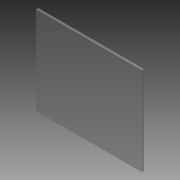
# Autodesk Inventor part: Wheel Shields
Saved by Autodesk Inventor 2013 (Build 170138000, 138)
## iProperties
Created: 2013-03-21
Part Number: Wheel Shields
Material: Polycarbonate, Clear
Document SubType Name: Modeling
Designer: actoennies
Mass: 73.7418 g
Surface Area: 404.838 cm^2
Volume: 61.4515 cm^3
Density: 1.2 g/cm^3
Author: actoennies
Autodesk Inventor part; units mm, degrees
ref_plane "YZ Plane" through (0, 0, 0) normal (1, 0, 0) x (0, 1, 0)
ref_plane "XZ Plane" through (0, 0, 0) normal (0, 1, 0) x (-1, 0, 0)
ref_plane "XY Plane" through (0, 0, 0) normal (0, 0, 1) x (1, 0, 0)
sketch "Sketch1" plane through (0, 0, 0) normal (0, 0, 1) x (1, 0, 0)
  line L0 (0, 0) -> (0, 127)
  line L1 (0, 127) -> (152.4, 127)
  line L2 (152.4, 127) -> (152.4, 0)
  line L3 (152.4, 0) -> (0, 0)
  dimension "d0" = 127
  dimension "d1" = 152.4
  constraints: 8 end point, 2 perpendicular, 1 parallel, 1 vertical
  measures "d0" distance of L0.start L0.end
  measures "d1" distance of L0.end L1.end
extrude "Extrusion1" add sketch "Sketch1" along normal blind 3.175
body "Solid1"
